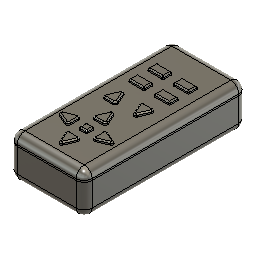
northreach_1_v3 (Autodesk Fusion 360 design; units mm, degrees)
Autodesk Fusion 360 part; units mm, degrees
sketch "Base" plane through (0, 0, 0) normal (0, 1, 0) x (1, 0, 0) in component "MainBody"
  line L0 (23.5, 51) -> (23.5, -51)
  line L1 (23.5, -51) -> (-23.5, -51)
  line L2 (22.5, -50) -> (-22.5, -50)
  line L3 (-22.5, 50) -> (22.5, 50)
  line L4 (22.5, 50) -> (-22.5, -50) construction
  line L5 (-23.5, 51) -> (23.5, -51) construction
  line L6 (-23.5, 51) -> (23.5, 51)
  line L7 (23.5, 51) -> (-23.5, -51) construction
  line L8 (-22.5, -50) -> (-22.5, 50)
  line L9 (-23.5, -51) -> (-23.5, 51)
  line L10 (22.5, 50) -> (22.5, -50)
  line L11 (-22.5, 50) -> (22.5, -50) construction
  dimension "d1" = 45
  dimension "d2" = 100
  dimension "d3" = 47
  dimension "d4" = 102
  constraint horizontal L3
  constraint perpendicular L3 L10
  constraint parallel L2 L3
  constraint parallel L8 L10
  constraint coincident origin L11
  constraint coincident origin L4
  constraint horizontal L6
  constraint perpendicular L0 L6
  constraint parallel L1 L6
  constraint parallel L0 L9
  constraint coincident origin L5
  constraint coincident origin L7
  measures "d1" distance of L2.start L2.end
  measures "d2" distance of L3.end L2.start
  measures "d3" distance of L1.end L0.end
  measures "d4" distance of L0.start L0.end
extrude "Extrude1" add sketch "Base" along normal blind 3 contours L2 L3 L8 L10 makes body 1 in component "MainBody"
extrude "Extrude2" add sketch "Base" along normal blind 20 bodies 1 in component "MainBody"
fillet "Fillet1" radius 5 2 edges at (-23.5, 0, 0) (23.5, 0, 0) on bodies 1 in component "MainBody"
fillet "Fillet1" radius 2 2 edges at (-22.5, 3, 0) (22.5, 3, 0) on bodies 1 in component "MainBody"
fillet "Fillet2" radius 5 10 edges at (-21.9142, 3.5858, -50) (0, 3, -50) (21.9142, 3.5858, -50) (21.9142, 3.5858, 50) (0, 3, 50) (-21.9142, 3.5858, 50) (-22.5, 12.5, 50) (22.5, 12.5, 50) (22.5, 12.5, -50) (-22.5, 12.5, -50) on bodies 1 in component "MainBody"
fillet "Fillet2" radius 5 10 edges at (23.5, 12.5, 51) (22.0355, 1.4645, 51) (0, 0, 51) (-22.0355, 1.4645, 51) (-23.5, 12.5, 51) (-23.5, 12.5, -51) (-22.0355, 1.4645, -51) (0, 0, -51) (22.0355, 1.4645, -51) (23.5, 12.5, -51) on bodies 1 in component "MainBody"
sketch "Base (2)" plane through (0, 3, 0) normal (0, 1, 0) x (-1, 0, 0) in component "TopCover"
  line L0 (20.5, 45) -> (-20.5, 45)
  line L1 (-20.5, 45) -> (-20.5, -45)
  line L2 (-20.5, -45) -> (20.5, -45)
  line L3 (20.5, -45) -> (20.5, 45)
  line L4 (48.5, 49) -> (91.5, -49) construction
  line L5 (85, 49) -> (85, 50)
  line L6 (85, 50) -> (55, 50)
  line L7 (91.5, 39.9985) -> (92.475, 39.9985)
  line L8 (46.5, 51) -> (93.5, 51)
  line L9 (91.5, -40) -> (92.475, -40)
  line L10 (55, 50) -> (55, 49)
  line L11 (55, 49) -> (85, 49)
  line L12 (47.5, 39.9985) -> (48.5, 39.9985)
  line L13 (91.5, 49) -> (48.5, -49) construction
  line L14 (93.5, -51) -> (46.5, -51)
  line L15 (48.5, 49) -> (91.5, 49)
  line L16 (85, -49) -> (85, -50)
  line L17 (55, -50) -> (55, -49)
  line L18 (92.475, -40) -> (92.475, 39.9985)
  line L19 (46.5, -51) -> (46.5, 51)
  line L20 (55, -49) -> (85, -49)
  line L21 (47.5, 39.9985) -> (47.5, -40)
  line L22 (93.5, 51) -> (93.5, -51)
  line L23 (91.5, -49) -> (48.5, -49)
  line L24 (46.5, 51) -> (93.5, -51) construction
  line L25 (91.5, 49) -> (91.5, -49)
  line L26 (91.5, 50) -> (91.5, -49)
  line L27 (93.5, 51) -> (46.5, -51) construction
  line L28 (48.5, -49) -> (48.5, 49)
  line L29 (47.5, -40) -> (48.5, -40)
  line L30 (85, -50) -> (55, -50)
  dimension "d17" = 47
  dimension "d18" = 102
  dimension "d19" = 43
  dimension "d20" = 98
  constraint horizontal L8
  constraint perpendicular L8 L22
  constraint parallel L8 L14
  constraint parallel L19 L22
  constraint horizontal L15
  constraint perpendicular L15 L25
  constraint parallel L15 L23
  constraint parallel L25 L28
  constraint vertical L21
  constraint vertical L18
  constraint vertical L26
  constraint coincident L12.start L21
  constraint coincident L29.start L21
  constraint coincident L9.start L26
  constraint coincident L9.end L18
  constraint perpendicular L9 L18
  constraint coincident L7.start L25
  constraint coincident L7.end L18
  constraint perpendicular L7 L18
  constraint horizontal L11
  constraint vertical L5
  constraint horizontal L6
  constraint vertical L10
  constraint coincident L10.end L15
  constraint horizontal L20
  constraint vertical L16
  constraint horizontal L30
  constraint vertical L17
  constraint coincident L17.end L23
  measures "d17" distance of L14.start L14.end
  measures "d18" distance of L8.end L14.start
  measures "d19" distance of L4.end L13.end
  measures "d20" distance of L4.end L13.start
extrude "Extrude1'" add sketch "Base (2)" along normal blind 2 separate body contours L11 L15 L20 L23 L25 L26 L28 makes body 2 in component "TopCover"
extrude "Extrude2'" add sketch "Base (2)" along normal blind 6 contours L8 L14 L19 L22 bodies 2 in component "TopCover"
extrude "Extrude3" add sketch "Base (2)" along normal blind 8.5 contours L5 L6 L10 L11 L15 | L7 L9 L18 L25 L26 | L12 L21 L28 L29 | L16 L17 L20 L23 L30 bodies 2 in component "TopCover"
fillet "Fillet1'" radius 5 2 edges at (-93.5, 3, 0) (-46.5, 3, 0) on bodies 2 in component "TopCover"
fillet "Fillet1'" radius 3.5 2 edges at (-91.5, 5, 0) (-48.5, 5, 0) on bodies 2 in component "TopCover"
fillet "Fillet2'" radius 5 10 edges at (-46.5, 8.5, 51) (-47.9645, 4.4645, 51) (-70, 3, 51) (-92.0355, 4.4645, 51) (-93.5, 8.5, 51) (-93.5, 8.5, -51) (-92.0355, 4.4645, -51) (-70, 3, -51) (-47.9645, 4.4645, -51) (-46.5, 8.5, -51) on bodies 2 in component "TopCover"
move_body "Move1" bodies 2 to x (-1, 0, 0) y (0, -1, 0) z (0, 0, 1) at (-140, 20.5, 0) in component "TopCover"
sketch "ButtonHoles" plane through (0, 17.5, 0) normal (0, 1, 0) x (-1, 0, 0) in component "TopCover"
  line L0 (51.5, -46) -> (88.5, -46)
  line L1 (88.5, -46) -> (88.5, 46)
  line L2 (88.5, 46) -> (51.5, 46)
  line L3 (51.5, 46) -> (51.5, -46)
  line L4 (83, -13.75) -> (83, -18.25)
  arc A0 (71.1295, 10.0141) -> (68.8705, 10.0141) centre (70, 10.4982) cw
  line L5 (66.1237, 16.4233) -> (68.8705, 10.0141)
  arc A1 (83, -13.75) -> (82.25, -13) centre (82.25, -13.75) ccw
  line L6 (57.75, -13) -> (66.25, -13)
  line L7 (78, -14) -> (78, -18)
  line L8 (59.4931, -5.0384) -> (64.5069, -5.0384)
  line L9 (80.5069, 4.1923) -> (75.4931, 4.1923)
  arc A2 (73, -18.25) -> (73.75, -19) centre (73.75, -18.25) ccw
  line L10 (64, -16) -> (60, -16)
  arc A3 (72.5069, 18.5) -> (73.8763, 16.4233) centre (72.5069, 17.0102) cw
  arc A4 (80.5069, 4.1923) -> (81.8763, 2.1156) centre (80.5069, 2.7025) cw
  line L11 (80, -16) -> (76, -16)
  line L12 (62, -0.423) -> (78, -0.423)
  arc A5 (74.1237, 2.1156) -> (75.4931, 4.1923) centre (75.4931, 2.7025) cw
  arc A6 (57.75, -13) -> (57, -13.75) centre (57.75, -13.75) ccw
  line L13 (72.5, 23.5) -> (67.5, 28.5) construction
  line L14 (71.1295, 10.0141) -> (73.8763, 16.4233)
  arc A7 (73.75, -13) -> (73, -13.75) centre (73.75, -13.75) ccw
  line L15 (70, 42.7307) -> (70, 33.5)
  arc A8 (66.1237, 16.4233) -> (67.4931, 18.5) centre (67.4931, 17.0102) cw
  arc A9 (73.8763, 35.5767) -> (72.5069, 33.5) centre (72.5069, 34.9898) cw
  arc A10 (73.75, -25) -> (73, -25.75) centre (73.75, -25.75) ccw
  arc A11 (79.5767, 22.1237) -> (77.5, 23.4931) centre (78.9898, 23.4931) cw
  line L16 (65.8763, -2.9617) -> (63.1295, 3.4475)
  arc A12 (66.25, -31) -> (67, -30.25) centre (66.25, -30.25) ccw
  arc A13 (60.8705, 3.4475) -> (63.1295, 3.4475) centre (62, 2.9635) cw
  arc A14 (67, -25.75) -> (66.25, -25) centre (66.25, -25.75) ccw
  arc A15 (60.8705, 3.4475) -> (63.1295, 3.4475) centre (62, 2.9635) cw
  line L17 (82.25, -31) -> (73.75, -31)
  line L18 (71.75, 28.5) -> (68.25, 28.5)
  line L19 (65.8763, -2.9617) -> (63.1295, 3.4475)
  line L20 (73.75, -25) -> (82.25, -25)
  arc A16 (73, -30.25) -> (73.75, -31) centre (73.75, -30.25) ccw
  line L21 (60.8705, 3.4475) -> (58.1237, -2.9617)
  line L22 (68.8705, 41.9859) -> (66.1237, 35.5767)
  line L23 (83, -25.75) -> (83, -30.25)
  arc A17 (60.4233, 29.8763) -> (62.5, 28.5069) centre (61.0102, 28.5069) cw
  line L24 (60.8705, 3.4475) -> (58.1237, -2.9617)
  line L25 (73, -25) -> (83, -31) construction
  line L26 (62.5, 23.4931) -> (62.5, 28.5069)
  line L27 (73, -30.25) -> (73, -25.75)
  arc A18 (67.5, 24.25) -> (68.25, 23.5) centre (68.25, 24.25) ccw
  line L28 (73, -18.25) -> (73, -13.75)
  line L29 (59.4931, -5.0384) -> (64.5069, -5.0384)
  arc A19 (59.4931, -5.0384) -> (58.1237, -2.9617) centre (59.4931, -3.5486) cw
  line L30 (62, 4.1923) -> (62, -5.0384)
  line L31 (57, -18.25) -> (57, -13.75)
  line L32 (62, 4.1923) -> (62, -5.0384)
  line L33 (73.75, -13) -> (82.25, -13)
  line L34 (67, -16) -> (73, -16)
  line L35 (67, -13.75) -> (67, -18.25)
  line L36 (79.1295, -4.2936) -> (81.8763, 2.1156)
  line L37 (62, -14) -> (62, -18)
  arc A20 (65.8763, -2.9617) -> (64.5069, -5.0384) centre (64.5069, -3.5486) cw
  arc A21 (65.8763, -2.9617) -> (64.5069, -5.0384) centre (64.5069, -3.5486) cw
  arc A22 (59.4931, -5.0384) -> (58.1237, -2.9617) centre (59.4931, -3.5486) cw
  arc A23 (67, -13.75) -> (66.25, -13) centre (66.25, -13.75) ccw
  line L38 (78, -5.0384) -> (78, 4.1923)
  arc A24 (79.1295, -4.2936) -> (76.8705, -4.2936) centre (78, -3.8095) cw
  line L39 (74.1237, 2.1156) -> (76.8705, -4.2936)
  line L40 (66.25, -31) -> (57.75, -31)
  line L41 (57, -30.25) -> (57, -25.75)
  line L42 (66.25, -19) -> (57.75, -19)
  arc A25 (57, -30.25) -> (57.75, -31) centre (57.75, -30.25) ccw
  arc A26 (57.75, -25) -> (57, -25.75) centre (57.75, -25.75) ccw
  line L43 (67, -25) -> (57, -31) construction
  line L44 (57, -25) -> (67, -31) construction
  line L45 (57.75, -25) -> (66.25, -25)
  line L46 (64, -28) -> (60, -28)
  line L47 (70, 9.2693) -> (70, 18.5)
  line L48 (68.25, 23.5) -> (71.75, 23.5)
  line L49 (80, -28) -> (76, -28)
  line L50 (54.0141, 24.8705) -> (60.4233, 22.1237)
  arc A27 (83, -25.75) -> (82.25, -25) centre (82.25, -25.75) ccw
  arc A28 (68.25, 28.5) -> (67.5, 27.75) centre (68.25, 27.75) ccw
  line L51 (83, -25) -> (73, -31) construction
  line L52 (53.2693, 26) -> (62.5, 26)
  line L53 (60.4233, 29.8763) -> (54.0141, 27.1295)
  line L54 (57, -13) -> (67, -19) construction
  arc A29 (82.25, -31) -> (83, -30.25) centre (82.25, -30.25) ccw
  line L55 (67.5, 27.75) -> (67.5, 24.25)
  arc A30 (67.4931, 33.5) -> (66.1237, 35.5767) centre (67.4931, 34.9898) cw
  line L56 (62, -26) -> (62, -30)
  arc A31 (54.0141, 24.8705) -> (54.0141, 27.1295) centre (54.4981, 26) cw
  arc A32 (62.5, 23.4931) -> (60.4233, 22.1237) centre (61.0102, 23.4931) cw
  line L57 (78, -26) -> (78, -30)
  line L58 (67, -28) -> (73, -28)
  line L59 (83, -13) -> (73, -19) construction
  line L60 (67, -13) -> (57, -19) construction
  line L61 (67, -25.75) -> (67, -30.25)
  arc A33 (57, -18.25) -> (57.75, -19) centre (57.75, -18.25) ccw
  line L62 (82.25, -19) -> (73.75, -19)
  arc A34 (68.8705, 41.9859) -> (71.1295, 41.9859) centre (70, 41.5019) cw
  arc A35 (82.25, -19) -> (83, -18.25) centre (82.25, -18.25) ccw
  line L63 (86.7307, 26) -> (77.5, 26)
  line L64 (67.5, 23.5) -> (72.5, 28.5) construction
  line L65 (72.5069, 18.5) -> (67.4931, 18.5)
  line L66 (77.5, 28.5069) -> (77.5, 23.4931)
  arc A36 (77.5, 28.5069) -> (79.5767, 29.8763) centre (78.9898, 28.5069) cw
  arc A37 (66.25, -19) -> (67, -18.25) centre (66.25, -18.25) ccw
  arc A38 (72.5, 27.75) -> (71.75, 28.5) centre (71.75, 27.75) ccw
  line L67 (73, -13) -> (83, -19) construction
  line L68 (72.5, 24.25) -> (72.5, 27.75)
  line L69 (73.8763, 35.5767) -> (71.1295, 41.9859)
  line L70 (67.4931, 33.5) -> (72.5069, 33.5)
  arc A39 (71.75, 23.5) -> (72.5, 24.25) centre (71.75, 24.25) ccw
  line L71 (85.9859, 27.1295) -> (79.5767, 29.8763)
  arc A40 (85.9859, 27.1295) -> (85.9859, 24.8705) centre (85.5019, 26) cw
  line L72 (79.5767, 22.1237) -> (85.9859, 24.8705)
  point P0 (70, 13.8847)
  point P1 (62, -28)
  point P2 (70, 18.5)
  point P3 (78, -16)
  point P4 (70, 38.1153)
  point P5 (77.5, 26)
  point P6 (82.1153, 26)
  point P7 (62.5, 26)
  point P8 (78, -0.423)
  point P9 (57.8847, 26)
  point P10 (57.8847, 26)
  point P11 (78, 4.1923)
  point P12 (62, -5.0384)
  point P13 (70.0007, -10.4459)
  point P14 (62, -16)
  point P15 (78, -0.423)
  point P16 (82.1153, 26)
  point P17 (59.5, -12)
  point P18 (62, -16)
  point P19 (59.5, -24)
  point P20 (62, -28)
  point P21 (70, -16)
  point P22 (62, -0.423)
  point P23 (70, -28)
  point P24 (78, -16)
  point P25 (70, 26)
  point P26 (78, -28)
  point P27 (70, 13.8847)
  point P28 (78, -28)
  point P29 (57.8847, 26)
  point P30 (82.1153, 26)
  point P31 (70, -0.423)
  point P32 (70, 33.5)
  point P33 (70, 13.8847)
  point P34 (62, -0.423)
  point P35 (62, -5.0384)
  point P36 (62, -0.423)
  point P37 (70, 38.1153)
  point P38 (70, 38.1153)
  dimension "d50" = 3
  dimension "d52" = 3
  dimension "d46" = 3
  dimension "d48" = 3
  dimension "d55" = 0.75
  dimension "d56" = 10
  dimension "d57" = 6
  dimension "d58" = 10
  dimension "d59" = 6
  dimension "d60" = 6
  dimension "d61" = 0.75
  dimension "d62" = 10
  dimension "d63" = 6
  dimension "d64" = 10
  dimension "d65" = 6
  dimension "d66" = 6
  dimension "d67" = 0.75
  dimension "d68" = 5
  constraint perpendicular L48 L68
  constraint parallel L18 L48
  constraint parallel L55 L68
  constraint coincident P25 L64
  constraint coincident P25 L13
  constraint coincident L64.end L18
  constraint coincident L64.end L68
  constraint tangent L18 A38
  constraint tangent A38 L68
  constraint coincident L13.end L18
  constraint coincident L13.end L55
  constraint tangent L18 A28
  constraint tangent A28 L55
  constraint equal A28 A38
  constraint coincident L64.start L55
  constraint coincident L64.start L48
  constraint tangent A18 L55
  constraint tangent A18 L48
  constraint equal A18 A38
  constraint coincident L13.start L48
  constraint coincident L13.start L68
  constraint tangent L48 A39
  constraint tangent L68 A39
  constraint equal A38 A39
  constraint tangent L8 A20
  constraint tangent L16 A20
  constraint tangent L8 A19
  constraint tangent L21 A19
  constraint tangent L16 A15
  constraint tangent A15 L21
  constraint midpoint P35 L8
  constraint midpoint L30.start A15
  constraint coincident P35 P12
  constraint perpendicular L8 L30
  constraint midpoint P36 L30
  constraint perpendicular L4 L33
  constraint parallel L33 L62
  constraint parallel L4 L28
  constraint perpendicular L6 L35
  constraint parallel L6 L42
  constraint parallel L31 L35
  constraint midpoint P21 L34
  constraint tangent A6 L31
  constraint tangent L6 A6
  constraint tangent L31 A33
  constraint tangent L42 A33
  constraint equal A6 A33
  constraint coincident L34.start L35
  constraint tangent L42 A37
  constraint tangent L35 A37
  constraint equal A6 A37
  constraint tangent L6 A23
  constraint tangent L35 A23
  constraint equal A6 A23
  constraint coincident L34.end L28
  constraint coincident L67.start L28
  constraint tangent A7 L33
  constraint tangent A7 L28
  constraint equal A6 A7
  constraint coincident L59.end L28
  constraint tangent A2 L28
  constraint tangent A2 L62
  constraint equal A2 A6
  constraint coincident L67.end L62
  constraint tangent L62 A35
  constraint tangent L4 A35
  constraint equal A6 A35
  constraint tangent A1 L33
  constraint tangent L4 A1
  constraint equal A1 A6
  constraint perpendicular L20 L23
  constraint parallel L17 L20
  constraint parallel L23 L27
  constraint perpendicular L45 L61
  constraint parallel L40 L45
  constraint parallel L41 L61
  constraint midpoint P23 L58
  constraint tangent L41 A26
  constraint tangent A26 L45
  constraint tangent L41 A25
  constraint tangent L40 A25
  constraint equal A25 A26
  constraint coincident L58.start L61
  constraint tangent A12 L40
  constraint tangent A12 L61
  constraint equal A12 A26
  constraint tangent A14 L45
  constraint tangent A14 L61
  constraint equal A14 A26
  constraint coincident L58.end L27
  constraint coincident L25.start L27
  constraint tangent A10 L20
  constraint tangent A10 L27
  constraint equal A10 A26
  constraint coincident L51.end L27
  constraint tangent A16 L27
  constraint tangent L17 A16
  constraint equal A16 A26
  constraint coincident L25.end L17
  constraint tangent L17 A29
  constraint tangent L23 A29
  constraint equal A26 A29
  constraint tangent L20 A27
  constraint tangent L23 A27
  constraint equal A26 A27
  constraint midpoint P18 L10
  constraint midpoint P24 L11
  constraint midpoint P20 L46
  constraint midpoint P28 L49
  constraint coincident P36 P34
  constraint tangent L29 A21
  constraint tangent L19 A21
  constraint tangent L29 A22
  constraint tangent L24 A22
  constraint tangent A13 L19
  constraint tangent A13 L24
  constraint midpoint P35 L29
  constraint midpoint L30.start A13
  constraint perpendicular L29 L32
  constraint midpoint P36 L32
  constraint tangent L9 A5
  constraint tangent A5 L39
  constraint tangent L9 A4
  constraint tangent A4 L36
  constraint tangent A24 L39
  constraint tangent L36 A24
  constraint midpoint P11 L9
  constraint midpoint L38.start A24
  constraint coincident P11 L38.end
  constraint perpendicular L9 L38
  constraint midpoint P15 L38
  constraint coincident P15 P8
  constraint tangent A8 L65
  constraint tangent L5 A8
  constraint tangent A3 L65
  constraint tangent A3 L14
  constraint tangent A0 L5
  constraint tangent A0 L14
  constraint midpoint P2 L65
  constraint midpoint L47.start A0
  constraint coincident P2 L47.end
  constraint perpendicular L47 L65
  constraint midpoint P33 L47
  constraint coincident P33 P27
  constraint tangent A11 L66
  constraint tangent A11 L72
  constraint tangent L66 A36
  constraint tangent A36 L71
  constraint tangent A40 L72
  constraint tangent L71 A40
  constraint midpoint P5 L66
  constraint midpoint L63.start A40
  constraint coincident P5 L63.end
  constraint perpendicular L63 L66
  constraint midpoint P30 L63
  constraint coincident P30 P16
  constraint tangent A17 L26
  constraint tangent A17 L53
  constraint tangent L26 A32
  constraint tangent L50 A32
  constraint tangent L53 A31
  constraint tangent L50 A31
  constraint midpoint P7 L26
  constraint midpoint L52.start A31
  constraint coincident P7 L52.end
  constraint perpendicular L26 L52
  constraint midpoint P29 L52
  constraint coincident P29 P10
  constraint tangent A9 L70
  constraint tangent A9 L69
  constraint tangent A30 L70
  constraint tangent L22 A30
  constraint tangent A34 L69
  constraint tangent L22 A34
  constraint midpoint P32 L70
  constraint midpoint L15.start A34
  constraint coincident P32 L15.end
  constraint perpendicular L15 L70
  constraint midpoint P38 L15
  constraint coincident P38 P37
  measures "d55" radius of A38
  measures "d56" distance of L67.end L59.end
  measures "d57" distance of L67.end L59.start
  measures "d58" distance of L60.end L54.end
  measures "d59" distance of L60.start L54.end
  measures "d60" distance of L28 L35
  measures "d61" radius of A6
  measures "d62" distance of L51.end L25.end
  measures "d63" distance of L51.start L25.end
  measures "d64" distance of L44.end L43.end
  measures "d65" distance of L44.end L43.start
  measures "d66" distance of L27 L61
  measures "d67" radius of A26
  measures "d68" distance of L18 L70
extrude "Extrude4" cut sketch "ButtonHoles" against normal blind 18 contours L4 A1 A2 A7 L28 L33 L62 A35 | A0 A3 L14 L47 L65 | A0 L5 A8 L47 L65 | L6 A6 L31 L35 A23 L42 A33 A37 | L8 A13 A15 L21 L24 L29 A19 L30 L32 A22 | L8 L12 L16 L19 L29 L30 L32 A20 A21 | L12 L16 A13 A15 L19 L30 L32 | L9 A4 L36 L38 A24 | L9 L12 A5 L38 L39 | L12 L38 A24 L39 | L15 A9 A34 L69 L70 | L15 L22 A30 A34 L70 | A10 L17 L20 A16 L23 L27 A27 A29 | A11 L63 L66 A40 L72 | L63 L66 A36 L71 A40 | A12 A14 L40 L41 A25 A26 L45 L61 | L18 A18 L48 A28 L55 A38 L68 A39 | A17 L26 L52 L53 A31 | L26 L50 L52 A31 A32 bodies 2 in component "TopCover"
sketch "Base (3)" plane through (0, 0, 0) normal (0, 1, 0) x (1, 0, 0) in component "TriangleButton"
  line L0 (47.0141, -44.1295) -> (53.4233, -46.8763)
  arc A0 (55.5, -45.5069) -> (53.4233, -46.8763) centre (54.0102, -45.5069) cw
  arc A1 (53.4233, -39.1237) -> (55.5, -40.4931) centre (54.0102, -40.4931) cw
  arc A2 (47.0141, -44.1295) -> (47.0141, -41.8705) centre (47.4981, -43) cw
  line L1 (55.5, -45.5069) -> (55.5, -40.4931)
  line L2 (53.4233, -39.1237) -> (47.0141, -41.8705)
  line L3 (53.4824, -39.2616) -> (47.0732, -42.0084)
  arc A3 (47.0732, -42.0084) -> (47.0732, -43.9916) centre (47.4981, -43) ccw
  line L4 (47.0732, -43.9916) -> (53.4824, -46.7384)
  arc A4 (53.4824, -46.7384) -> (55.35, -45.5069) centre (54.0102, -45.5069) ccw
  line L5 (55.35, -45.5069) -> (55.35, -40.4931)
  arc A5 (55.35, -40.4931) -> (53.4824, -39.2616) centre (54.0102, -40.4931) ccw
  point P0 (55.5, -43)
  point P1 (50.8847, -43)
  point P2 (50.8847, -43)
  point P3 (50.8847, -43)
  dimension "d107" = 0.15
  constraint tangent A1 L1
  constraint tangent A1 L2
  constraint tangent A0 L1
  constraint tangent L0 A0
  constraint tangent A2 L2
  constraint tangent L0 A2
  constraint midpoint P0 L1
  constraint coincident P2 P1
extrude "Extrude1''" add sketch "Base (3)" along normal blind 8 separate body contours L3 A3 L4 A4 L5 A5 makes body 3 in component "TriangleButton"
ref_plane "WorkPlane1" through (50.8847, 4, 43) normal (0, 1, 0) x (1, 0, 0) in component "TriangleButton"
sketch "Lip" plane through (0, 4, 0) normal (0, 1, 0) x (1, 0, 0) in component "TriangleButton"
  line L0 (55.35, -45.5069) -> (55.35, -40.4931)
  arc A0 (55.35, -40.4931) -> (53.4824, -39.2616) centre (54.0102, -40.4931) ccw
  line L1 (53.4824, -39.2616) -> (47.0732, -42.0084)
  arc A1 (53.4824, -46.7384) -> (55.35, -45.5069) centre (54.0102, -45.5069) ccw
  arc A2 (47.0732, -42.0084) -> (47.0732, -43.9916) centre (47.4981, -43) ccw
  line L2 (47.0732, -43.9916) -> (53.4824, -46.7384)
  arc A3 (56.35, -40.4931) -> (53.0885, -38.3424) centre (54.0102, -40.4931) ccw
  line L3 (53.0885, -38.3424) -> (46.6793, -41.0893)
  arc A4 (46.6793, -41.0893) -> (46.6793, -44.9107) centre (47.4981, -43) ccw
  line L4 (46.6793, -44.9107) -> (53.0885, -47.6576)
  arc A5 (53.0885, -47.6576) -> (56.35, -45.5069) centre (54.0102, -45.5069) ccw
  line L5 (56.35, -45.5069) -> (56.35, -40.4931)
  dimension "d108" = 1
extrude "Extrude2''" add sketch "Lip" along normal mid plane 1 bodies 3 in component "TriangleButton"
sketch "Base (4)" plane through (0, 0, 0) normal (0, 1, 0) x (1, 0, 0) in component "SquareButton"
  line L0 (51.25, -20.5) -> (54.75, -20.5)
  line L1 (55.5, -19.75) -> (55.5, -16.25)
  line L2 (50.5, -16.25) -> (50.5, -19.75)
  arc A0 (50.5, -19.75) -> (51.25, -20.5) centre (51.25, -19.75) ccw
  line L3 (54.75, -15.5) -> (51.25, -15.5)
  arc A1 (51.25, -15.5) -> (50.5, -16.25) centre (51.25, -16.25) ccw
  arc A2 (55.5, -16.25) -> (54.75, -15.5) centre (54.75, -16.25) ccw
  line L4 (55.5, -15.5) -> (50.5, -20.5) construction
  arc A3 (54.75, -20.5) -> (55.5, -19.75) centre (54.75, -19.75) ccw
  line L5 (50.5, -15.5) -> (55.5, -20.5) construction
  line L6 (51.25, -20.35) -> (54.75, -20.35)
  arc A4 (54.75, -20.35) -> (55.35, -19.75) centre (54.75, -19.75) ccw
  line L7 (55.35, -19.75) -> (55.35, -16.25)
  arc A5 (55.35, -16.25) -> (54.75, -15.65) centre (54.75, -16.25) ccw
  line L8 (54.75, -15.65) -> (51.25, -15.65)
  arc A6 (51.25, -15.65) -> (50.65, -16.25) centre (51.25, -16.25) ccw
  line L9 (50.65, -16.25) -> (50.65, -19.75)
  arc A7 (50.65, -19.75) -> (51.25, -20.35) centre (51.25, -19.75) ccw
  point P0 (53, -18)
  dimension "d77" = 0.75
  dimension "d111" = -0.15
  constraint horizontal L3
  constraint perpendicular L2 L3
  constraint parallel L0 L3
  constraint parallel L1 L2
  constraint coincident P0 L4
  constraint coincident P0 L5
  constraint coincident L4.end L0
  constraint coincident L4.end L2
  constraint tangent L0 A0
  constraint tangent L2 A0
  constraint coincident L5.end L0
  constraint coincident L5.end L1
  constraint tangent L0 A3
  constraint tangent L1 A3
  constraint equal A0 A3
  constraint coincident L4.start L1
  constraint coincident L4.start L3
  constraint tangent L1 A2
  constraint tangent L3 A2
  constraint equal A0 A2
  constraint coincident L5.start L3
  constraint coincident L5.start L2
  constraint tangent L3 A1
  constraint tangent L2 A1
  constraint equal A0 A1
  measures "d77" radius of A0
extrude "Extrude1'''" add sketch "Base (4)" along normal blind 8 separate body contours L6 A4 L7 A5 L8 A6 L9 A7 makes body 4 in component "SquareButton"
ref_plane "WorkPlane1" through (53, 4, 18) normal (0, 1, 0) x (1, 0, 0) in component "SquareButton"
sketch "Lip (2)" plane through (0, 4, 0) normal (0, 1, 0) x (1, 0, 0) in component "SquareButton"
  line L0 (54.75, -15.65) -> (51.25, -15.65)
  arc A0 (55.35, -16.25) -> (54.75, -15.65) centre (54.75, -16.25) ccw
  line L1 (55.35, -19.75) -> (55.35, -16.25)
  arc A1 (51.25, -15.65) -> (50.65, -16.25) centre (51.25, -16.25) ccw
  line L2 (50.65, -16.25) -> (50.65, -19.75)
  arc A2 (50.65, -19.75) -> (51.25, -20.35) centre (51.25, -19.75) ccw
  line L3 (51.25, -20.35) -> (54.75, -20.35)
  arc A3 (54.75, -20.35) -> (55.35, -19.75) centre (54.75, -19.75) ccw
  arc A4 (49.65, -19.75) -> (51.25, -21.35) centre (51.25, -19.75) ccw
  line L4 (51.25, -21.35) -> (54.75, -21.35)
  arc A5 (54.75, -21.35) -> (56.35, -19.75) centre (54.75, -19.75) ccw
  line L5 (56.35, -19.75) -> (56.35, -16.25)
  arc A6 (56.35, -16.25) -> (54.75, -14.65) centre (54.75, -16.25) ccw
  line L6 (54.75, -14.65) -> (51.25, -14.65)
  arc A7 (51.25, -14.65) -> (49.65, -16.25) centre (51.25, -16.25) ccw
  line L7 (49.65, -16.25) -> (49.65, -19.75)
  dimension "d112" = 1
extrude "Extrude2'''" add sketch "Lip (2)" along normal mid plane 1 bodies 4 in component "SquareButton"
sketch "Base (5)" plane through (0, 0, 0) normal (0, 1, 0) x (1, 0, 0) in component "RectangleButton"
  line L0 (48, 3) -> (58, 9) construction
  arc A0 (48.75, 9) -> (48, 8.25) centre (48.75, 8.25) ccw
  line L1 (53, 4) -> (53, 8)
  line L2 (57.25, 3) -> (48.75, 3)
  arc A1 (58, 8.25) -> (57.25, 9) centre (57.25, 8.25) ccw
  line L3 (48.75, 9) -> (57.25, 9)
  line L4 (48, 3.75) -> (48, 8.25)
  line L5 (58, 3) -> (48, 9) construction
  line L6 (58, 8.25) -> (58, 3.75)
  line L7 (51, 6) -> (55, 6)
  arc A2 (48, 3.75) -> (48.75, 3) centre (48.75, 3.75) ccw
  arc A3 (57.25, 3) -> (58, 3.75) centre (57.25, 3.75) ccw
  arc A4 (48.15, 3.75) -> (48.75, 3.15) centre (48.75, 3.75) ccw
  line L8 (57.25, 3.15) -> (48.75, 3.15)
  arc A5 (57.25, 3.15) -> (57.85, 3.75) centre (57.25, 3.75) ccw
  line L9 (57.85, 8.25) -> (57.85, 3.75)
  arc A6 (57.85, 8.25) -> (57.25, 8.85) centre (57.25, 8.25) ccw
  line L10 (48.75, 8.85) -> (57.25, 8.85)
  arc A7 (48.75, 8.85) -> (48.15, 8.25) centre (48.75, 8.25) ccw
  line L11 (48.15, 3.75) -> (48.15, 8.25)
  point P0 (58, 6)
  point P1 (53, 6)
  point P2 (53, 6)
  dimension "d86" = 10
  dimension "d87" = 6
  dimension "d115" = 0.15
  constraint horizontal L2
  constraint perpendicular L2 L4
  constraint parallel L2 L3
  constraint parallel L4 L6
  constraint coincident P0 L6
  constraint coincident L5.start L6
  constraint tangent L2 A3
  constraint tangent L6 A3
  constraint coincident L0.end L6
  constraint tangent A1 L6
  constraint tangent A1 L3
  constraint coincident L5.end L3
  constraint tangent A0 L3
  constraint tangent A0 L4
  constraint tangent L2 A2
  constraint tangent L4 A2
  constraint midpoint P2 L7
  measures "d86" distance of L0.end L5.end
  measures "d87" distance of L0.start L5.end
extrude "Extrude1''''" add sketch "Base (5)" along normal blind 8 separate body contours A4 L8 A5 L9 A6 L10 A7 L11 makes body 5 in component "RectangleButton"
ref_plane "WorkPlane1" through (53, 4, -6) normal (0, 1, 0) x (1, 0, 0) in component "RectangleButton"
sketch "Lip (3)" plane through (0, 4, 0) normal (0, 1, 0) x (1, 0, 0) in component "RectangleButton"
  line L0 (57.85, 3.75) -> (57.85, 8.25)
  arc A0 (57.85, 8.25) -> (57.25, 8.85) centre (57.25, 8.25) ccw
  line L1 (57.25, 8.85) -> (48.75, 8.85)
  arc A1 (57.25, 3.15) -> (57.85, 3.75) centre (57.25, 3.75) ccw
  line L2 (48.75, 3.15) -> (57.25, 3.15)
  arc A2 (48.15, 3.75) -> (48.75, 3.15) centre (48.75, 3.75) ccw
  line L3 (48.15, 8.25) -> (48.15, 3.75)
  arc A3 (48.75, 8.85) -> (48.15, 8.25) centre (48.75, 8.25) ccw
  line L4 (57.25, 9.85) -> (48.75, 9.85)
  arc A4 (48.75, 9.85) -> (47.15, 8.25) centre (48.75, 8.25) ccw
  line L5 (47.15, 8.25) -> (47.15, 3.75)
  arc A5 (47.15, 3.75) -> (48.75, 2.15) centre (48.75, 3.75) ccw
  line L6 (48.75, 2.15) -> (57.25, 2.15)
  arc A6 (57.25, 2.15) -> (58.85, 3.75) centre (57.25, 3.75) ccw
  line L7 (58.85, 3.75) -> (58.85, 8.25)
  arc A7 (58.85, 8.25) -> (57.25, 9.85) centre (57.25, 8.25) ccw
  dimension "d116" = 1
extrude "Extrude2''''" add sketch "Lip (3)" along normal mid plane 1 bodies 5 in component "RectangleButton"
fillet "Fillet1''" radius 0.75 8 edges at (53, 8, -3.15) (57.6743, 8, -3.3257) (57.85, 8, -6) (57.6743, 8, -8.6743) (53, 8, -8.85) (48.3257, 8, -8.6743) (48.15, 8, -6) (48.3257, 8, -3.3257) on bodies 5 in component "RectangleButton"
fillet "Fillet1'''" radius 0.75 8 edges at (53, 8, 15.65) (50.8257, 8, 15.8257) (50.65, 8, 18) (50.8257, 8, 20.1743) (53, 8, 20.35) (55.1743, 8, 20.1743) (55.35, 8, 18) (55.1743, 8, 15.8257) on bodies 4 in component "SquareButton"
fillet "Fillet1''''" radius 0.75 6 edges at (50.2778, 8, 40.635) (46.4193, 8, 43) (50.2778, 8, 45.365) (54.7477, 8, 46.6255) (55.35, 8, 43) (54.7477, 8, 39.3745) on bodies 3 in component "TriangleButton"
component "MainBody" placed x (1, 0, 0) y (0, 1, 0) z (0, 0, 1) at (0, 0, 0)
component "TopCover" placed x (1, 0, 0) y (0, 1, 0) z (0, 0, 1) at (70, 8.5, 0)
component "TriangleButton" placed x (1, 0, 0) y (0, 1, 0) z (0, 0, 1) at (-63, 19.5, -17)
component "SquareButton" placed x (1, 0, 0) y (0, 1, 0) z (0, 0, 1) at (-53, 19.5, 8)
component "RectangleButton" placed x (1, 0, 0) y (0, 1, 0) z (0, 0, 1) at (-45, 19.5, -10)
component "TriangleButton" placed x (0, 0, -1) y (0, 1, 0) z (1, 0, 0) at (-43, 19.5, 89)
component "TriangleButton" placed x (-1, 0, 0) y (0, 1, 0) z (0, 0, -1) at (63, 19.5, 69)
component "TriangleButton" placed x (0, 0, 1) y (0, 1, 0) z (-1, 0, 0) at (43, 19.5, -37)
component "TriangleButton" placed x (0, 0, 1) y (0, 1, 0) z (-1, 0, 0) at (35, 19.5, -51.3077)
component "TriangleButton" placed x (0, 0, -1) y (0, 1, 0) z (1, 0, 0) at (-35, 19.5, 50.4616)
component "RectangleButton" placed x (1, 0, 0) y (0, 1, 0) z (0, 0, 1) at (-61, 19.5, -10)
component "RectangleButton" placed x (1, 0, 0) y (0, 1, 0) z (0, 0, 1) at (-45, 19.5, -22)
component "RectangleButton" placed x (1, 0, 0) y (0, 1, 0) z (0, 0, 1) at (-61, 19.5, -22)
equation "d51 = '3'"
equation "d53 = '4'"
equation "d47 = '1'"
equation "d49 = '2'"
named bodies: "MainBody", "TopCover", "TriangleButton", "SquareButton", "RectangleButton"
